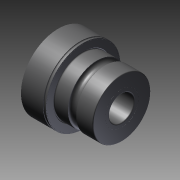
# Autodesk Inventor part: NKXZ9
Saved by Autodesk Inventor 2011 SP1 (Build 150282100, 282)
## iProperties
Created: 2016-11-09
Part Number: NKXZ9
Catalog Web Link: www.cadenas.de
Description: NKXZ-Needle Roller Bearings with Thrust Ball Bearings - With Inner Ring
Vendor: MISUMI
Document SubType Name: Modeling
Designer: psAdmin
Manufacturer: MISUMI
Mass: 7.94497 g
Surface Area: 35.7401 cm^2
Volume: 7.94497 cm^3
Density: 1 g/cm^3
Category: PARTsolutions
Company: MISUMI
Title: NKXZ9
Author: Cadenas PARTsolutions
Comments: Needle Roller Bearings with Thrust Ball Bearings - With Inner Ring
PSOL_IDENT_0: {$CADENAS_DATA\23d-libs\misumi\metric\12_bearing_holders\nkxz.prj},150 {VTYP=3D},{NB=NKXZ9},{LINA=NK
PSOL_IDENT_1: XZ9},{NN=NKXZ},{DATE=17.06.2016 05:47:22},{GEOMDATE=25.02.2016 05:06:56},{VERSION=},{LINEID=20},{LIN
PSOL_IDENT_2: ESUBID=-1},{WBVAR=}  {NB=NKXZ9},{LINA=NKXZ9},{KT=DUMMY},{PN=NKXZ9},{TYPE=NKXZ},{DD=9},{D=21},{B=16},
PSOL_IDENT_3: {L=23},{T=9},{RR=0.3},{RR1=0.3},{DD1=12},{D1=27.0},{LL=6.5},{AA=21.7}
NN: NKXZ
NT: Needle Roller Bearings with Thrust Ball Bearings - With Inner Ring
NB: NKXZ9
NBSYN: $PN.
LINA: NKXZ9
PN: NKXZ9
DD: 9
D: 21
B: 16
L: 23
T: 9
RR: 0.3
RR1: 0.3
DD1: 12
D1: 27.0
LL: 6.5
AA: 21.7
SUPPLIER: MISUMI
ARTICLENO: NKXZ9
BOMINFO: NKXZ9
CREATOR: CADENAS GmbH
Autodesk Inventor part; units mm, degrees
ref_plane "YZ Plane" through (0, 0, 0) normal (1, 0, 0) x (0, 1, 0)
ref_plane "XZ Plane" through (0, 0, 0) normal (0, 1, 0) x (-1, 0, 0)
ref_plane "XY Plane" through (0, 0, 0) normal (0, 0, 1) x (1, 0, 0)
sketch "Sketch_1" plane through (0, 0, 0) normal (0, 0, 1) x (1, 0, 0)
  line L0 (23, 0) -> (0, 0)
  line L1 (0, 13.5) -> (0, 10.87)
  arc A0 (0, 10.83) -> (0, 10.87) centre (0, 10.85) ccw
  line L2 (0, 10.83) -> (0, 6.3)
  arc A1 (0, 6.3) -> (0.3, 6) centre (0.3, 6.3) ccw
  line L3 (0.3, 6) -> (7, 6)
  line L4 (7, 6) -> (7, 4.5)
  line L5 (7, 4.5) -> (22.7, 4.5)
  arc A2 (22.7, 4.5) -> (23, 4.8) centre (22.7, 4.8) ccw
  line L6 (23, 4.8) -> (23, 5.98)
  arc A3 (23, 6.02) -> (23, 5.98) centre (23, 6) ccw
  line L7 (23, 6.02) -> (23, 10.2)
  arc A4 (23, 10.2) -> (22.7, 10.5) centre (22.7, 10.2) ccw
  line L8 (22.7, 10.5) -> (17, 10.5)
  arc A5 (14, 10.5) -> (17, 10.5) centre (15.5, 10.5) ccw
  line L9 (14, 10.5) -> (9.3, 10.5)
  arc A6 (9, 10.8) -> (9.3, 10.5) centre (9, 10.5) ccw
  line L10 (9, 10.8) -> (9, 13.18)
  arc A7 (9, 13.22) -> (9, 13.18) centre (9, 13.2) ccw
  line L11 (9, 13.22) -> (9, 13.5)
  line L12 (9, 13.5) -> (8.55, 13.5)
  arc A8 (7.95, 13.5) -> (8.55, 13.5) centre (8.25, 13.5) ccw
  line L13 (7.95, 13.5) -> (0, 13.5)
  constraints: 28 end point, 18 point on circle, 9 centre point
revolve "Revolution1" add sketch "Sketch_1" angle 360 about axis through (23, 0, 0) along (1, 0, 0)
ref_plane "to_housing_XY" through (9, 0, 0) normal (1, 0, 0) x (0, 0, -1)
ref_plane "to_housing_YZ" through (9, 0, 0) normal (0, 0, -1) x (0, 1, 0)
ref_plane "to_housing_ZX" through (9, 0, 0) normal (0, 1, 0) x (1, 0, 0)
body "Solid1"
